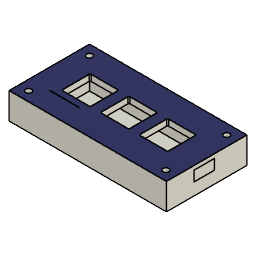
assembled-model.STEP (Autodesk Fusion 360 design; units mm, degrees)
part number: 2026-06-17-19-48-32-750
Autodesk Fusion 360 part; units mm, degrees
sketch "Sketch1" plane through (0, 0, 0) normal (0, 0, 1) x (1, 0, 0)
  line L0 (0, 20) -> (57.4, 20)
  line L1 (57.4, 20) -> (57.4, 0.4)
  line L2 (57.4, 0.4) -> (0, 0.4)
  line L3 (0, 0.4) -> (0, 20)
  line L4 (-10, 30) -> (67.4, 30)
  line L5 (67.4, 30) -> (67.4, -9.6)
  line L6 (67.4, -9.6) -> (-10, -9.6)
  line L7 (-10, -9.6) -> (-10, 30)
  circle A0 centre (-5, 25) radius 1.45
  circle A1 centre (-5, -4.9) radius 1.45
  circle A2 centre (62.4768, -4.9) radius 1.45
  circle A3 centre (62.4768, 25) radius 1.45
  dimension "d1" = 57.4
  dimension "d2" = 19.6
  dimension "d3" = 77.4
  dimension "d4" = 39.6
  dimension "d5" = 2.9
  dimension "d6" = 2.9
  dimension "d7" = 2.9
  dimension "d8" = 2.9
  constraint horizontal L0
  constraint vertical L1
  constraint horizontal L2
  constraint vertical L3
  constraint horizontal L4
  constraint vertical L5
  constraint horizontal L6
  constraint vertical L7
  measures "d1" distance of L0.start L0.end
  measures "d2" distance of L0.start L2.end
  measures "d3" distance of L4.start L4.end
  measures "d4" distance of L4.start L6.end
  measures "d5" diameter of A0
  measures "d6" diameter of A1
  measures "d7" diameter of A2
  measures "d8" diameter of A3
extrude "Extrude1" add sketch "Sketch1" along normal blind 3 contours L0 L1 L2 L3 | L4 L5 L6 L7 makes body 1
extrude "Extrude2" add sketch "Sketch1" along normal blind 10 bodies 1
sketch "plate-2026-06-17T15_17_22.943Z" plane through (0, 0, 3) normal (0, 0, 1) x (1, 0, 0)
  line L0 (3.325, 17.475, 7) -> (16.325, 17.475, 7)
  line L1 (3.325, 3.475, 7) -> (16.325, 3.475, 7)
  line L2 (2.825, 16.975, 7) -> (2.825, 3.975, 7)
  line L3 (16.825, 16.975, 7) -> (16.825, 3.975, 7)
  arc A0 through (3.325, 17.475, 7) (2.9714, 17.3286, 7) (2.825, 16.975, 7)
  arc A1 through (16.825, 16.975, 7) (16.6786, 17.3286, 7) (16.325, 17.475, 7)
  arc A2 through (2.825, 3.975, 7) (2.9714, 3.6214, 7) (3.325, 3.475, 7)
  arc A3 through (16.325, 3.475, 7) (16.6786, 3.6214, 7) (16.825, 3.975, 7)
  line L4 (22.375, 17.475, 7) -> (35.375, 17.475, 7)
  line L5 (22.375, 3.475, 7) -> (35.375, 3.475, 7)
  line L6 (21.875, 16.975, 7) -> (21.875, 3.975, 7)
  line L7 (35.875, 16.975, 7) -> (35.875, 3.975, 7)
  arc A4 through (22.375, 17.475, 7) (22.0214, 17.3286, 7) (21.875, 16.975, 7)
  arc A5 through (35.875, 16.975, 7) (35.7286, 17.3286, 7) (35.375, 17.475, 7)
  arc A6 through (21.875, 3.975, 7) (22.0214, 3.6214, 7) (22.375, 3.475, 7)
  arc A7 through (35.375, 3.475, 7) (35.7286, 3.6214, 7) (35.875, 3.975, 7)
  line L8 (41.425, 17.475, 7) -> (54.425, 17.475, 7)
  line L9 (41.425, 3.475, 7) -> (54.425, 3.475, 7)
  line L10 (40.925, 16.975, 7) -> (40.925, 3.975, 7)
  line L11 (54.925, 16.975, 7) -> (54.925, 3.975, 7)
  arc A8 through (41.425, 17.475, 7) (41.0714, 17.3286, 7) (40.925, 16.975, 7)
  arc A9 through (54.925, 16.975, 7) (54.7786, 17.3286, 7) (54.425, 17.475, 7)
  arc A10 through (40.925, 3.975, 7) (41.0714, 3.6214, 7) (41.425, 3.475, 7)
  arc A11 through (54.425, 3.475, 7) (54.7786, 3.6214, 7) (54.925, 3.975, 7)
  line L12 (0, 0.5329, 7) -> (58, 0, 7)
  line L13 (0, 20, 7) -> (57.45, 20, 7)
  line L14 (0, 0.5329, 7) -> (0, 20, 7)
  line L15 (58, 0, 7) -> (57.45, 20, 7)
extrude "Extrude3" add sketch "plate-2026-06-17T15_17_22.943Z" 1 faces at (38.2923, -3.5528, 10) along normal blind 3 contours L12 L13 L14 L15 in plane through (0, 0, 10) normal (0, 0, 1) on bodies 1 bodies 1
sketch "Sketch3" plane through (67.4, 0, 0) normal (1, 0, 0) x (0, 1, 0)
  line L0 (-9.6, 0) -> (30, 0)
  line L1 (30, 0) -> (30, 13)
  line L2 (30, 13) -> (-9.6, 13)
  line L3 (-9.6, 13) -> (-9.6, 0)
  line L4 (4, 11) -> (14, 11)
  line L5 (14, 11) -> (14, 6)
  line L6 (14, 6) -> (4, 6)
  line L7 (4, 6) -> (4, 11)
  dimension "d16" = 10
  dimension "d17" = 5
  constraint horizontal L4
  constraint vertical L5
  constraint horizontal L6
  constraint vertical L7
  measures "d16" distance of L4.start L4.end
  measures "d17" distance of L4.start L6.end
surface "Extrude4" add extruded along (1, 0, 0) between 0 and -10 profiles "Sketch3" section 1 contours L4 L5 L6 L7 separate body makes body 2
